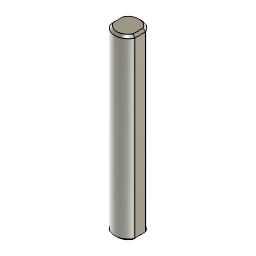
仮シャフト (Autodesk Fusion 360 design; units mm, degrees)
Autodesk Fusion 360 part; units mm, degrees
sketch "スケッチ1" plane through (0, 0, 0) normal (0, 0, 1) x (1, 0, 0)
  line L0 (5.5, 0) -> (-5.5, 0)
  line L1 (-5.5, 0) -> (-5.5, 2.3979)
  line L2 (-5.5, -2.3979) -> (-5.5, 0)
  line L3 (5.4842, -2.4339) -> (5.4842, 2.4339)
  arc A0 (5.4842, 2.4339) -> (-5.5, 2.3979) centre (0, 0) ccw
  arc A1 (-5.5, -2.3979) -> (5.4842, -2.4339) centre (0, 0) ccw
  dimension "d1" = 12
  constraint coincident A0.centre A1.centre
  constraint horizontal L0
  constraint perpendicular L0 L1
  constraint coincident L2.start A0
  constraint perpendicular L0 L2
  constraint perpendicular L0 L3
  constraint concentric A0 A1
  measures "d1" diameter of A0
extrude "押し出し1" add sketch "スケッチ1" along normal blind 80
chamfer "面取り1" distance 1 angle 45 2 faces at (-0.0118, -2, 80) (-0.0118, -2, 0)
